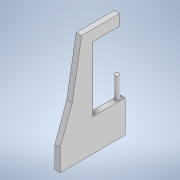
# Autodesk Inventor part: Pala1
Saved by Autodesk Inventor 2020.3 (Build 243373000, 373)
## iProperties
Created: 2021-03-12
Part Number: Pala1
Material: Generic
Document SubType Name: Modeling
Designer: alexo
Density: 1 g/cm^3
Appearance: Default
Author: alexo
Autodesk Inventor part; units mm, degrees
ref_plane "YZ Plane" through (0, 0, 0) normal (1, 0, 0) x (0, 1, 0)
ref_plane "XZ Plane" through (0, 0, 0) normal (0, 1, 0) x (-1, 0, 0)
ref_plane "XY Plane" through (0, 0, 0) normal (0, 0, 1) x (1, 0, 0)
sketch "Sketch1" plane through (0, 0, 0) normal (1, 0, 0) x (0, 1, 0)
  line L0 (-21.3033, 45) -> (-41.466, 45)
  line L1 (-41.466, 45) -> (-41.466, -15)
  line L2 (-41.466, -15) -> (-11.466, -15)
  line L3 (-11.466, -15) -> (-11.466, 15)
  line L4 (-11.466, 15) -> (48.534, 15)
  line L5 (48.534, 15) -> (48.534, -10)
  line L6 (48.534, -10) -> (58.534, -10)
  line L7 (58.534, -10) -> (58.534, 25.2188)
  line L8 (58.534, 25.2188) -> (9.0933, 33.9365)
  line L9 (9.0933, 33.9365) -> (-21.3033, 45)
  point P0 (0, 0)
  dimension "d0" = 60
  dimension "d1" = 30
  dimension "d2" = 30
  dimension "d3" = 60
  dimension "d4" = 10
  dimension "d5" = 100
  dimension "d7" = 25
  dimension "d8" = 160
  dimension "d9" = 58.534
  dimension "d10" = 10
  dimension "d11" = 35
  dimension "d12" = 35
  constraints: 20 end point, 3 parallel, 2 perpendicular, 2 vertical, 1 horizontal
  measures "d0" distance between parallel lines of L3 L5
  measures "d1" distance of L2.end L3.end
  measures "d2" distance between parallel lines of L3 L1
  measures "d3" distance between parallel lines of L2 L0
  measures "d4" distance between parallel lines of L5 L7
  measures "d5" angle of L7 L8
  measures "d7" distance of L4.end L5.end
  measures "d8" angle of L0 L9
  measures "d9" distance from line of point (0, 0) L7
  measures "d10" distance from line of point (0, 0) L6
  measures "d11" distance from line of point (0, 0) L8
  measures "d12" distance from line of point (0, 0) L9
extrude "Extrusion1" add sketch "Sketch1" along normal blind 5
sketch "Sketch2" plane through (0, -11.466, 15) normal (0, 1, 0) x (1, 0, 0)
  circle A0 centre (2.4001, 25) radius 2
  line L0 (0, 30) -> (0, 0) projected
  line L1 (0, 0) -> (5, 0) projected
  line L2 (5, 30) -> (5, 0) projected
  line L3 (0, 30) -> (5, 30) projected
  point P0 (0, 15)
  dimension "d15" = 4
  dimension "d16" = 25
  constraints: 1 centre point
  measures "d15" diameter of A0
  measures "d16" distance from line of L1 A0.centre
extrude "Extrusion2" add sketch "Sketch2" along normal blind 20 contours A0
body "Solid1"
